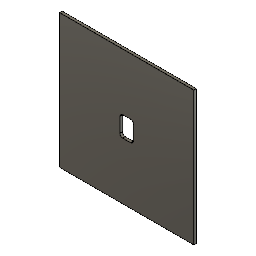
Table_17p1_Problem_12 (Autodesk Fusion 360 design; units mm, degrees)
Autodesk Fusion 360 part; units mm, degrees
sketch "Sketch1" plane through (0, 0, 0) normal (0, 0, 1) x (1, 0, 0)
  line L0 (-250, 250) -> (250, 250)
  line L1 (250, 250) -> (250, -250)
  line L2 (250, -250) -> (-250, -250)
  line L3 (-250, -250) -> (-250, 250)
  line L4 (-15, 37.5) -> (15, 37.5)
  line L5 (25, 27.5) -> (25, -27.5)
  line L6 (15, -37.5) -> (-15, -37.5)
  line L7 (-25, -27.5) -> (-25, 27.5)
  line L8 (0, 250) -> (0, -250) construction
  line L9 (-250, 0) -> (250, 0) construction
  arc A0 (-15, 37.5) -> (-25, 27.5) centre (-15, 27.5) ccw
  arc A1 (25, 27.5) -> (15, 37.5) centre (15, 27.5) ccw
  arc A2 (15, -37.5) -> (25, -27.5) centre (15, -27.5) ccw
  arc A3 (-25, -27.5) -> (-15, -37.5) centre (-15, -27.5) ccw
  line L10 (0, 37.5) -> (0, -37.5) construction
  line L11 (-25, 0) -> (25, 0) construction
  point P0 (-25, 37.5)
  point P1 (25, 37.5)
  point P2 (-25, -37.5)
  dimension "Total_Width" = 500
  dimension "Hole_Width" = 50
  dimension "Hole_Height" = 75
  dimension "Fillet_Radius" = 10
  constraint horizontal L0
  constraint vertical L1
  constraint horizontal L2
  constraint vertical L3
  constraint horizontal L4
  constraint vertical L5
  constraint horizontal L6
  constraint vertical L7
  constraint midpoint L0 L8.start
  constraint midpoint L2 L8.end
  constraint midpoint L3 L9.start
  constraint midpoint L1 L9.end
  constraint equal L0 L3
  constraint coincident L9 origin
  constraint coincident origin L8
  constraint coincident P0 L4
  constraint coincident P0 L7
  constraint tangent L4 A0
  constraint tangent L7 A0
  constraint coincident P1 L4
  constraint coincident P1 L5
  constraint tangent L4 A1
  constraint tangent L5 A1
  constraint equal A0 A1
  constraint tangent L5 A2
  constraint tangent L6 A2
  constraint equal A0 A2
  constraint coincident P2 L6
  constraint coincident P2 L7
  constraint tangent L6 A3
  constraint tangent L7 A3
  constraint equal A0 A3
  constraint midpoint L4 L10.start
  constraint midpoint L6 L10.end
  constraint midpoint L7 L11.start
  constraint midpoint L5 L11.end
  constraint coincident origin L11
  constraint coincident origin L10
  measures "Total_Width" distance of L0.start L0.end
  measures "Hole_Width" distance of P0 P1
  measures "Hole_Height" distance of P0 P2
  measures "Fillet_Radius" radius of A0
extrude "Extrude1" add sketch "Sketch1" along normal mid plane 10
equation "Thickness = 1 cm"
